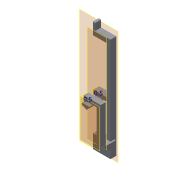
# Autodesk Inventor part: 08_Opentrons_Autofocus_flexurebaering
Saved by Autodesk Inventor 2019.4 (Build 234330000, 330)
## iProperties
Created: 2020-11-20
Part Number: 08_Opentrons_Autofocus_flexurebaering
Material: Generic
Document SubType Name: Modeling
Designer: diederichbenedict
Density: 1 g/cm^3
Appearance: Default
Author: diederichbenedict
Autodesk Inventor part; units mm, degrees
ref_plane "YZ Plane" through (0, 0, 0) normal (1, 0, 0) x (0, 1, 0)
ref_plane "XZ Plane" through (0, 0, 0) normal (0, 1, 0) x (-1, 0, 0)
ref_plane "XY Plane" through (0, 0, 0) normal (0, 0, 1) x (1, 0, 0)
ref_plane "Work Plane1" through (0, 0, 0) normal (0, 0, 1) x (1, 0, 0)
sketch "Sketch1" plane through (0, 0, 0) normal (0, 0, 1) x (1, 0, 0)
  line L0 (17.1585, 59.9787) -> (2.1585, 59.9787) construction
  line L1 (2.1585, 59.9787) -> (2.1585, 62.7008) construction
  line L2 (2.1585, 62.7008) -> (17.1585, 62.7008) construction
  line L3 (17.1585, 62.7008) -> (17.1585, 91.3397) construction
  line L4 (17.1585, 91.3397) -> (-18.8415, 91.3397) construction
  line L5 (-18.8415, 91.3397) -> (-18.8415, -14.6603) construction
  line L6 (-18.8415, -14.6603) -> (17.1585, -14.6603) construction
  line L7 (17.1585, -14.6603) -> (17.1585, 59.9787) construction
  line L8 (13.8585, 17.3397) -> (13.863, 4.6397) construction
  line L9 (13.863, 4.6397) -> (6.6783, 4.6397) construction
  arc A0 (-15.6915, 17.3397) -> (6.6783, 4.6397) centre (-0.9353, 17.2801) ccw construction
  arc A1 (6.6783, 30.0397) -> (-15.6915, 17.3397) centre (-0.9353, 17.3993) ccw construction
  line L10 (13.863, 30.0397) -> (6.6783, 30.0397) construction
  line L11 (13.8585, 17.3397) -> (13.863, 30.0397) construction
  circle A2 centre (-0.9353, 17.3993) radius 10.125 projected
  line L12 (17.1585, -14.6603) -> (-0.8415, -14.6603)
  line L13 (-0.8415, -14.6603) -> (-0.8415, -0.6603)
  line L14 (-0.8415, -0.6603) -> (17.1585, -0.6603)
  line L15 (17.1585, -0.6603) -> (17.1585, -14.6603)
  line L16 (17.1585, 0.8765) -> (13.1585, 0.8765)
  line L17 (13.1585, 0.8765) -> (13.1585, 91.3397)
  line L18 (13.1585, 91.3397) -> (17.1585, 91.3397)
  line L19 (17.1585, 91.3397) -> (17.1585, 0.8765)
  line L20 (13.1585, 34.2801) -> (-0.9353, 34.2801)
  line L21 (-0.9353, 34.2801) -> (-0.9353, 38.2801)
  line L22 (-0.9353, 38.2801) -> (13.1585, 38.2801)
  line L23 (13.1585, 38.2801) -> (13.1585, 34.2801)
  line L24 (13.1585, 91.3397) -> (-0.9353, 91.3397)
  line L25 (-0.9353, 91.3397) -> (-0.9353, 86.3397)
  line L26 (-0.9353, 86.3397) -> (13.1585, 86.3397)
  line L27 (13.1585, 86.3397) -> (13.1585, 91.3397)
  line L28 (-0.9353, 91.3397) -> (1.5647, 91.3397)
  line L29 (1.5647, 91.3397) -> (1.5647, 98.3397)
  line L30 (1.5647, 98.3397) -> (-0.9353, 98.3397)
  line L31 (-0.9353, 98.3397) -> (-0.9353, 91.3397)
  arc A3 (-5.6352, 28.9821) -> (3.1207, 29.223) centre (-0.9353, 17.3993) ccw projected
  arc A4 (-5.6352, 28.9821) -> (3.1207, 29.223) centre (-0.9353, 17.3993) ccw projected
  dimension "d18" = 18
  dimension "d19" = 14
  dimension "d20" = 4
  dimension "d21" = 4
  dimension "d37" = 5
  dimension "d38" = 2.5
  dimension "d39" = 7
  dimension "d41" = 17
  constraints: 40 end point, 10 parallel, 5 horizontal, 5 perpendicular, 3 point on line
  measures "d18" distance of L13.end L14.end
  measures "d19" distance of L12.end L13.end
  measures "d20" distance of L17.end L18.end
  measures "d21" distance of L20.end L21.end
  measures "d37" distance of L25.end L24.end
  measures "d38" distance of L30.end L29.end
  measures "d39" distance of L29.end L28.end
  measures "d41" distance from line of L20 A0.centre
extrude "Extrusion1" add sketch "Sketch1" along normal blind 6 contours L12 L13 L14 L15 | L16 L17 L18 L19 | L20 L21 L22 L17 | L17 L26 L25 L24 | L24 L31 L30 L29
ref_plane "Work Plane2" through (0, 0, 11) normal (0, 0, 1) x (1, 0, 0)
sketch "Sketch2" plane through (0, 0, 11) normal (0, 0, 1) x (1, 0, 0)
  line L0 (-0.9353, 34.2801) -> (13.1585, 34.2801) projected
  line L1 (13.1585, 34.2801) -> (13.1585, 0.8765) projected
  line L2 (13.1585, 0.8765) -> (17.1585, 0.8765) projected
  line L3 (17.1585, 0.8765) -> (17.1585, 91.3397) projected
  line L4 (17.1585, 91.3397) -> (1.5647, 91.3397) projected
  line L5 (13.1585, 86.3397) -> (13.1585, 38.2801) projected
  line L6 (13.1585, 38.2801) -> (-0.9353, 38.2801) projected
  line L7 (-0.9353, 38.2801) -> (-0.9353, 34.2801) projected
  line L8 (13.1585, 38.2801) -> (-0.9353, 38.2801) projected
  line L9 (13.1585, 38.2801) -> (17.1585, 38.2801)
  line L10 (17.1585, 91.3397) -> (1.5647, 91.3397) projected
  line L11 (13.1585, 91.3397) -> (-0.9353, 91.3397)
  line L12 (-0.9353, 91.3397) -> (-0.9353, 86.3397)
  line L13 (-0.9353, 86.3397) -> (13.1585, 86.3397)
  line L14 (13.1585, 86.3397) -> (13.1585, 91.3397)
  line L15 (-0.9353, 91.3397) -> (2.0647, 91.3397)
  line L16 (2.0647, 91.3397) -> (2.0647, 99.3397)
  line L17 (2.0647, 99.3397) -> (-0.9353, 99.3397)
  line L18 (-0.9353, 99.3397) -> (-0.9353, 91.3397)
  line L19 (-0.9353, 98.3397) -> (-0.9353, 86.3397) projected
  line L20 (-0.9353, 86.3397) -> (13.1585, 86.3397) projected
  line L21 (1.5647, 91.3397) -> (1.5647, 98.3397) projected
  line L22 (1.5647, 98.3397) -> (-0.9353, 98.3397) projected
  point P0 (0, 0)
  dimension "d34" = 5
  dimension "d35" = 3
  dimension "d36" = 8
  constraints: 18 end point, 4 parallel, 3 perpendicular, 2 horizontal, 1 point on line
  measures "d34" distance of L12.end L11.end
  measures "d35" distance of L17.end L16.end
  measures "d36" distance of L16.end L15.end
extrude "Extrusion2" add sketch "Sketch2" along normal blind 5 contours L7 L6 L9 L3 L2 L1 L0
sketch "Sketch3" plane through (17.1585, -14.6603, 0) normal (1, 0, 0) x (0, 0, -1)
  line L0 (0, 14) -> (0, 0) projected
  line L1 (0, 14) -> (-6, 14) projected
  line L2 (-6, 0) -> (-6, 14) projected
  line L3 (0, 0) -> (-6, 0) projected
  line L4 (0, 106) -> (0, 15.5368) projected
  line L5 (0, 106) -> (-6, 106) projected
  line L6 (-6, 15.5368) -> (-6, 106) projected
  line L7 (0, 15.5368) -> (-6, 15.5368) projected
  line L8 (-11, 15.5368) -> (-11, 52.9404) projected
  line L9 (-11, 52.9404) -> (-16, 52.9404) projected
  line L10 (-16, 15.5368) -> (-16, 52.9404) projected
  line L11 (-11, 15.5368) -> (-16, 15.5368) projected
  line L12 (-6, 14) -> (-6, 0) projected
  line L13 (-11.5, 14.0368) -> (-6, 14.0368)
  line L14 (-6, 14.0368) -> (-6, 9.0368)
  line L15 (-6, 9.0368) -> (-11.5, 9.0368)
  line L16 (-11.5, 9.0368) -> (-11.5, 14.0368)
  line L17 (-11, 15.5368) -> (-16, 15.5368) projected
  line L18 (-11, 15.5368) -> (-11.5, 15.5368)
  line L19 (-11.5, 15.5368) -> (-11.5, 14.0368)
  line L20 (-11.5, 14.0368) -> (-11, 14.0368)
  line L21 (-11, 14.0368) -> (-11, 15.5368)
  line L22 (0, 15.5368) -> (-0.5, 15.5368)
  line L23 (-0.5, 15.5368) -> (-0.5, 14)
  line L24 (-0.5, 14) -> (0, 14)
  line L25 (0, 14) -> (0, 15.5368)
  line L26 (-6, 15.5368) -> (-6, 106) projected
  line L27 (-6, 54.4404) -> (-11.5, 54.4404)
  line L28 (-11.5, 54.4404) -> (-11.5, 59.4404)
  line L29 (-11.5, 59.4404) -> (-6, 59.4404)
  line L30 (-6, 59.4404) -> (-6, 54.4404)
  line L31 (-11, 52.9404) -> (-16, 52.9404) projected
  line L32 (-11, 52.9404) -> (-11.5, 52.9404)
  line L33 (-11.5, 52.9404) -> (-11.5, 54.4404)
  line L34 (-11.5, 54.4404) -> (-11, 54.4404)
  line L35 (-11, 54.4404) -> (-11, 52.9404)
  point P0 (0, 14.6603)
  dimension "d25" = 5
  dimension "d26" = 0.5
  dimension "d27" = 0.5
  dimension "d28" = 5
  dimension "d29" = 0.5
  dimension "d30" = 1.5
  dimension "d31" = 1.5
  dimension "d40" = 0
  constraints: 40 end point, 10 parallel, 6 point on line, 5 horizontal, 5 perpendicular
  measures "d25" distance of L13.end L14.end
  measures "d26" distance of L20.end L19.end
  measures "d27" distance of L24.end L23.end
  measures "d28" distance of L27.end L28.end
  measures "d29" distance of L33.end L34.end
  measures "d30" distance between parallel lines of L27 L9
  measures "d31" distance between parallel lines of L13 L11
  measures "d40" distance between parallel lines of L33 L28
extrude "Extrusion3" add sketch "Sketch3" against normal up to surface (4 mm away) contours L1 L23 L7 L25 | L2 L15 L16 L13 L14 | L13 L19 L11 L21
ref_plane "Work Plane3" through (0, 0, 18) normal (0, 0, 1) x (1, 0, 0)
sketch "Sketch4" plane through (0, 0, 18) normal (0, 0, 1) x (1, 0, 0)
  line L0 (17.1585, 34.8891) -> (-18.8415, 34.8891)
  line L1 (-0.9353, 34.2801) -> (13.1585, 34.2801) projected
  line L2 (13.1585, 34.2801) -> (13.1585, 0.8765) projected
  line L3 (13.1585, 0.8765) -> (17.1585, 0.8765) projected
  line L4 (17.1585, 0.8765) -> (17.1585, 38.2801) projected
  line L5 (17.1585, 38.2801) -> (-0.9353, 38.2801) projected
  line L6 (-0.9353, 38.2801) -> (-0.9353, 34.2801) projected
  line L7 (-4.5265, 27.3641) -> (2.6559, 27.3641) projected
  arc A0 (9.49, 15.527) -> (2.6559, 27.3641) centre (-0.9353, 17.3993) ccw projected
  line L8 (9.49, 15.527) -> (5.8988, 9.3069) projected
  arc A1 (-7.7695, 9.3069) -> (5.8988, 9.3069) centre (-0.9353, 17.3993) ccw projected
  line L9 (-7.7695, 9.3069) -> (-11.3607, 15.527) projected
  arc A2 (-4.5265, 27.3641) -> (-11.3607, 15.527) centre (-0.9353, 17.3993) ccw projected
  arc A3 (-3.2146, 30.3993) -> (-4.8009, 29.6174) centre (-3.2146, 28.3993) ccw projected
  arc A4 (-5.6352, 28.9821) -> (-4.8009, 29.6174) centre (-6.3872, 30.8354) ccw projected
  arc A5 (-5.6352, 28.9821) -> (3.1207, 29.223) centre (-0.9353, 17.3993) ccw projected
  arc A6 (2.3012, 29.7571) -> (3.1207, 29.223) centre (3.7697, 31.1148) ccw projected
  arc A7 (2.3012, 29.7571) -> (0.8326, 30.3993) centre (0.8326, 28.3993) ccw projected
  line L10 (0.8326, 30.3993) -> (-3.2146, 30.3993) projected
  arc A8 (2.4113, 29.8589) -> (0.8326, 30.5493) centre (0.8326, 28.3993) ccw
  arc A9 (2.4113, 29.8589) -> (3.1694, 29.3649) centre (3.7697, 31.1148) ccw
  arc A10 (-5.6916, 29.1211) -> (3.1694, 29.3649) centre (-0.9353, 17.3993) ccw
  arc A11 (-5.6916, 29.1211) -> (-4.9199, 29.7087) centre (-6.3872, 30.8354) ccw
  arc A12 (-3.2146, 30.5493) -> (-4.9199, 29.7087) centre (-3.2146, 28.3993) ccw
  line L11 (-3.2146, 30.5493) -> (0.8326, 30.5493)
  line L12 (4.6209, 28.7638) -> (7.5318, 31.6747)
  line L13 (4.6209, 28.7638) -> (8.7375, 28.7638) construction
  line L14 (7.5318, 31.6747) -> (7.5318, 32.7801)
  line L15 (7.5318, 32.7801) -> (-0.9353, 32.7801)
  line L16 (-0.9353, 38.2801) -> (-0.9353, 34.2801) projected
  line L17 (-0.9353, 33.5573) -> (-0.9353, 30.5493)
  line L18 (-0.9353, 32.7801) -> (-0.9353, 30.5493)
  point P0 (0, 0)
  dimension "d43" = 0.15
  dimension "d44" = 45
  dimension "d49" = 1.5
  constraints: 16 end point, 11 point on circle, 5 centre point, 4 point on line, 2 horizontal, 2 vertical, 1 equal length, 1 perpendicular, 7 other
  measures "d43" radial gap between concentric circles of A7 A8
  measures "d44" angle of L13 L12
  measures "d49" distance between parallel lines of L1 L15
extrude "Extrusion4" add sketch "Sketch4" against normal up to surface (18 mm away) contours A8 L11 L17 L15 L14 L12 A10 A9
sketch "Sketch5" plane through (-0.9353, 30.5493, 18) normal (-1, 0, 0) x (0, 0, 1)
  line L0 (-7, 7.7307) -> (-7, 3.7307) projected
  line L1 (-7, 3.7307) -> (-2, 3.7307) projected
  line L2 (-2, 7.7307) -> (-2, 3.7307) projected
  line L3 (-7, 7.7307) -> (-2, 7.7307) projected
  line L4 (-18, 2.2307) -> (-18, 0) projected
  line L5 (0, 0) -> (-18, 0) projected
  line L6 (0, 2.2307) -> (0, 0) projected
  line L7 (0, 2.2307) -> (-18, 2.2307) projected
  line L8 (-18, 3.7307) -> (-18, 7.7307) projected
  line L9 (-18, 3.7307) -> (-12, 3.7307) projected
  line L10 (-12, 7.7307) -> (-12, 3.7307) projected
  line L11 (-18, 7.7307) -> (-12, 7.7307) projected
  line L12 (0, 2.2307) -> (-18, 2.2307) projected
  line L13 (-18, 3.7307) -> (-17.5, 3.7307)
  line L14 (-17.5, 3.7307) -> (-17.5, 2.2307)
  line L15 (-17.5, 2.2307) -> (-18, 2.2307)
  line L16 (-18, 2.2307) -> (-18, 3.7307)
  line L17 (-7, 3.7307) -> (-6.5, 3.7307)
  line L18 (-6.5, 3.7307) -> (-6.5, 2.2307)
  line L19 (-6.5, 2.2307) -> (-7, 2.2307)
  line L20 (-7, 2.2307) -> (-7, 3.7307)
  point P0 (-18, -30.5493)
  dimension "d47" = 0.5
  dimension "d48" = 0.5
  constraints: 16 end point, 4 parallel, 2 horizontal, 2 perpendicular, 2 point on line
  measures "d47" distance of L14.end L15.end
  measures "d48" distance of L18.end L19.end
sketch "Sketch7" plane through (-0.9353, 32.7801, 18) normal (0, 1, 0) x (1, 0, 0)
  circle A0 centre (-0.2556, 2.7408) radius 1.45 projected
  line L0 (-0.2556, 2.7408) -> (-0.2556, 15.61) construction
  line L1 (1.3944, 2.7408) -> (1.3944, 15.61)
  line L2 (-1.9056, 15.61) -> (-1.9056, 2.7408)
  arc A1 (-1.9056, 2.7408) -> (1.3944, 2.7408) centre (-0.2556, 2.7408) ccw
  arc A2 (1.3944, 15.61) -> (-1.9056, 15.61) centre (-0.2556, 15.61) ccw
  line L3 (-0.2556, 2.7408) -> (12.6135, 2.7408) construction
  point P0 (0.9353, 18)
  point P1 (-0.2556, 9.1754)
  dimension "d50" = 90
  dimension "d51" = 0.2
  constraints: 10 end point, 4 point on circle, 4 tangent, 2 centre point, 1 horizontal, 1 midpoint, 1 parallel, 1 perpendicular
  measures "d50" angle of L3 L0
  measures "d51" radial gap between concentric circles of A0 A1
extrude "Extrusion5" cut sketch "Sketch7" against normal blind 5 contours A0 | A1 L2 A2 L1
body "Solid1"
